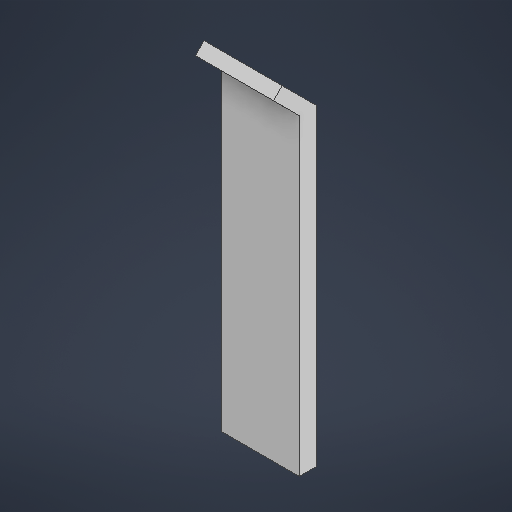
# Autodesk Inventor part: Soporte_Ultrasonido
Saved by Autodesk Inventor 2026 (Build 300175000, 175)
## iProperties
Created: 2025-06-27
Part Number: Soporte_Ultrasonido
Material: Genérico
Document SubType Name: Modeling
Designer: oscar
Density: 1 g/cm^3
Appearance: Valor por defecto
Author: oscar
Autodesk Inventor part; units mm, degrees
ref_plane "YZ Plane" through (0, 0, 0) normal (1, 0, 0) x (0, 1, 0)
ref_plane "XZ Plane" through (0, 0, 0) normal (0, 1, 0) x (-1, 0, 0)
ref_plane "XY Plane" through (0, 0, 0) normal (0, 0, 1) x (1, 0, 0)
sketch "Boceto6" plane through (0, 0, 0) normal (1, 0, 0) x (0, 1, 0)
  line L0 (0, 0) -> (180, 0)
  line L1 (180, 0) -> (180, -10)
  line L2 (180, -10) -> (0, -10)
  line L3 (0, -10) -> (0, 0)
  dimension "d12" = 180
  dimension "d13" = 10
  constraints: 8 end point, 2 parallel, 1 horizontal, 1 perpendicular
  measures "d12" distance of L1.end L2.end
  measures "d13" distance of L0.end L1.end
extrude "Extrusión3" add sketch "Boceto6" along normal mid plane 45
sketch "Boceto7" plane through (22.5, 0, 0) normal (1, 0, 0) x (0, 0, -1)
  line L0 (10, 0) -> (10, 180) projected
  line L1 (10, 180) -> (0, 180) projected
  line L2 (10, 180) -> (0, 180)
  line L3 (0, 180) -> (-14.8492, 194.8492)
  line L4 (10, 180) -> (-9.8492, 199.8492)
  line L5 (10, 180) -> (38.0711, 180) construction
  line L6 (-9.8492, 199.8492) -> (-14.8492, 194.8492)
  point P0 (0, 0)
  dimension "d16" = 21
  dimension "d17" = 135
  dimension "d18" = 135
  constraints: 10 end point, 2 horizontal, 1 equal length, 1 perpendicular
  measures "d16" distance of L1.end L3.end
  measures "d17" angle of L2 L3
  measures "d18" angle of L5 L4
extrude "Extrusión4" add sketch "Boceto7" against normal blind 45
sketch "Boceto8" plane through (22.5, 180, -10) normal (0, 0.7071068, -0.7071068) x (-1, 0, 0)
  circle A0 centre (10.275, 15) radius 8
  circle A1 centre (34.725, 15) radius 8
  line L0 (0, 0) -> (0, 28.0711) projected
  line L1 (45, 0) -> (0, 0) projected
  point P0 (22.5, -120.2082)
  dimension "d21" = 16
  dimension "d22" = 16
  dimension "d23" = 24.45
  dimension "d24" = 10.275
  dimension "d25" = 15
  dimension "d26" = 15
  constraints: 2 centre point
  measures "d21" diameter of A0
  measures "d22" diameter of A1
  measures "d23" distance of A0.centre A1.centre
  measures "d24" distance from line of L0 A0.centre
  measures "d25" distance from line of L1 A1.centre
  measures "d26" distance from line of L1 A0.centre
extrude "Extrusión5" cut sketch "Boceto8" against normal blind 8.25
